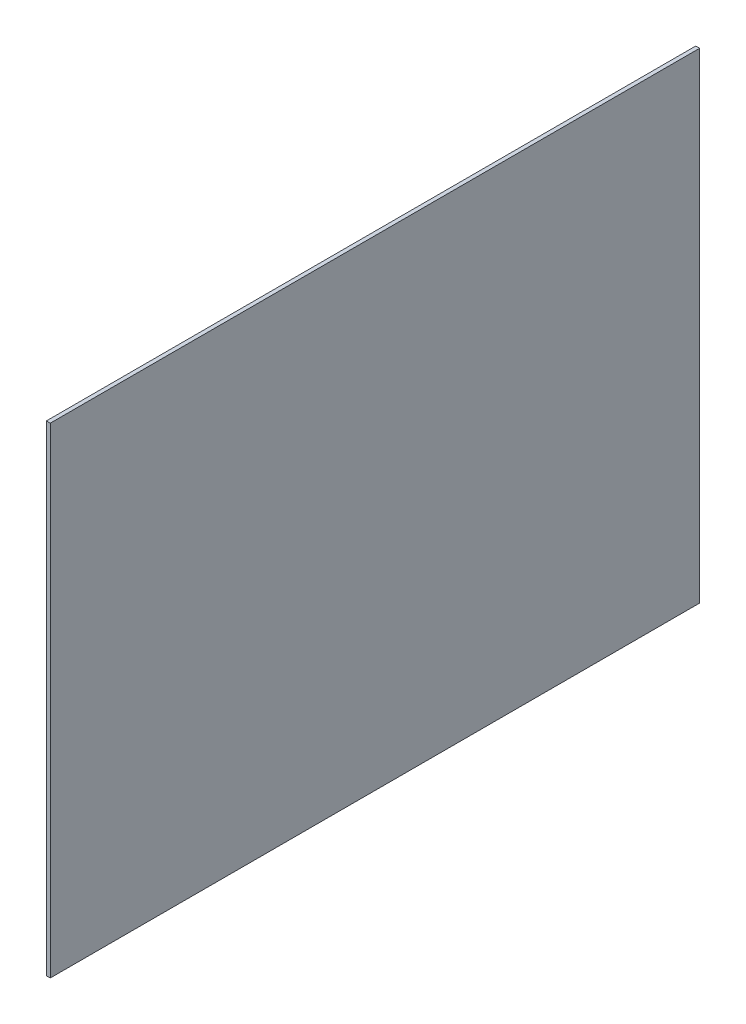
# Autodesk Inventor part: Width plate
Saved by Autodesk Inventor 2019.4 (Build 234330000, 330)
## iProperties
Created: 2019-12-06
Part Number: Width plate
Material: Polycarbonate, Clear
Document SubType Name: Modeling
Designer: Mark
Mass: 888 g
Surface Area: 3769.6 cm^2
Volume: 740 cm^3
Density: 1.2 g/cm^3
Appearance: Polycarbonate - Clear
Author: Mark
Autodesk Inventor part; units mm, degrees
ref_plane "YZ Plane" through (0, 0, 0) normal (1, 0, 0) x (0, 1, 0)
ref_plane "XZ Plane" through (0, 0, 0) normal (0, 1, 0) x (-1, 0, 0)
ref_plane "XY Plane" through (0, 0, 0) normal (0, 0, 1) x (1, 0, 0)
sketch "Sketch1" plane through (0, 0, 0) normal (1, 0, 0) x (0, 1, 0)
  line L0 (0, 0) -> (370, 0)
  line L1 (370, 0) -> (370, -500)
  line L2 (370, -500) -> (0, -500)
  line L3 (0, -500) -> (0, 0)
  dimension "d0" = 370
  dimension "d1" = 500
  constraints: 8 end point, 2 parallel, 1 horizontal, 1 perpendicular
  measures "d0" distance of L1.end L2.end
  measures "d1" distance of L0.end L1.end
extrude "Extrusion1" add sketch "Sketch1" along normal blind 3
body "Solid1"
